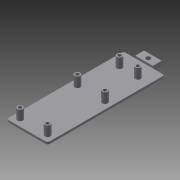
# Autodesk Inventor part: NodeMCU_MQ-7_bottom_v0.2
Saved by Autodesk Inventor 2014 SP1 (Build 180222100, 222)
## iProperties
Created: 2016-10-23
Part Number: NodeMCU_MQ-7_bottom_v0.2
Material: Generic
Document SubType Name: Modeling
Designer: danielsikar
Density: 1 g/cm^3
Appearance: Default
Author: danielsikar
Autodesk Inventor part; units mm, degrees
ref_plane "YZ Plane" through (0, 0, 0) normal (1, 0, 0) x (0, 1, 0)
ref_plane "XZ Plane" through (0, 0, 0) normal (0, 1, 0) x (-1, 0, 0)
ref_plane "XY Plane" through (0, 0, 0) normal (0, 0, 1) x (1, 0, 0)
sketch "Sketch3" plane through (0, 0, 0) normal (0, 0, 1) x (1, 0, 0)
  line L0 (0, 0) -> (37, 0)
  line L1 (37, 0) -> (37, 105.5)
  line L2 (37, 105.5) -> (0, 105.5)
  line L3 (0, 105.5) -> (0, 0)
  dimension "d5" = 37
  dimension "d6" = 105.5
  constraints: 8 end point, 2 parallel, 1 horizontal, 1 perpendicular
  measures "d5" distance of L2.end L1.end
  measures "d6" distance of L1.end L0.end
extrude "Extrusion2" add sketch "Sketch3" along normal blind 2
fillet "Fillet1" radius 2 4 edges at (0, 0, 1) (37, 0, 1) (37, 105.5, 1) (0, 105.5, 1)
sketch "Sketch5" plane through (0, 0, 2) normal (0, 0, 1) x (1, 0, 0)
  line L0 (2, 101.5) -> (2, 4) projected
  line L1 (4, 2) -> (33, 2) projected
  circle A0 centre (6.1, 6.1) radius 2.5
  circle A1 centre (6.1, 6.1) radius 1.5
  line L2 (0, 103.5) -> (0, 2) projected
  line L3 (2, 0) -> (35, 0) projected
  circle A2 centre (6.1, 57.9) radius 2.5
  circle A3 centre (6.1, 57.9) radius 1.5
  circle A4 centre (30.9, 6.1) radius 2.5
  circle A5 centre (30.9, 6.1) radius 1.5
  circle A6 centre (30.9, 57.9) radius 2.5
  circle A7 centre (30.9, 57.9) radius 1.5
  circle A8 centre (10.25, 91.7) radius 2.5
  circle A9 centre (10.25, 91.7) radius 1.5
  circle A10 centre (26.75, 91.7) radius 2.5
  circle A11 centre (26.75, 91.7) radius 1.5
  point P0 (0, 0)
  dimension "d15" = 5
  dimension "d16" = 3
  dimension "d17" = 6.1
  dimension "d18" = 6.1
  dimension "d21" = 51.8
  dimension "d24" = 24.8
  dimension "d27" = 5
  dimension "d28" = 33.8
  dimension "d29" = 4.15
  dimension "d30" = 3
  dimension "d31" = 5
  dimension "d32" = 16.5
  dimension "d33" = 3
  constraints: 12 centre point, 6 coincident, 1 horizontal, 1 vertical, 12 other
  measures "d15" diameter of A0
  measures "d16" diameter of A1
  measures "d17" distance from line of A1.centre L2
  measures "d18" distance from line of A0.centre L3
  measures "d21" distance of A0.centre A2.centre
  measures "d24" distance of A0.centre A4.centre
  measures "d27" diameter of A8
  measures "d28" vertical distance of A8.centre A2.centre
  measures "d29" horizontal distance of A8.centre A2.centre
  measures "d30" diameter of A9
  measures "d31" diameter of A10
  measures "d32" distance of A10.centre A8.centre
  measures "d33" diameter of A11
extrude "Extrusion4" add sketch "Sketch5" along normal blind 9
sketch "Sketch6" plane through (2, 105.5, 0) normal (0, 1, 0) x (1, 0, 0)
  line L0 (33, 0) -> (0, 0) projected
  line L1 (8.5, 0) -> (24.5, 0)
  line L2 (24.5, 0) -> (24.5, -4)
  line L3 (24.5, -4) -> (8.5, -4)
  line L4 (8.5, -4) -> (8.5, 0)
  line L5 (-2, 0) -> (-2, -2) projected
  point P0 (-2, -11)
  dimension "d37" = 16
  dimension "d38" = 4
  dimension "d39" = 10.5
  constraints: 8 end point, 2 parallel, 1 horizontal, 1 perpendicular, 1 point on line
  measures "d37" distance of L2.end L3.end
  measures "d38" distance of L1.end L2.end
  measures "d39" distance from line of L3.end L5
extrude "Extrusion5" add sketch "Sketch6" along normal blind 8
sketch "Sketch7" plane through (7.5, 105.5, 4) normal (0, 0, 1) x (1, 0, 0)
  circle A0 centre (11, 4) radius 2
  line L0 (3, 0) -> (3, 8) projected
  point P0 (-7.5, -105.5)
  point P1 (3, 5)
  point P2 (3, 3)
  dimension "d43" = 4
  dimension "d62" = 8
  constraints: 1 centre point
  measures "d43" diameter of A0
  measures "d62" distance from line of A0.centre L0
extrude "Extrusion6" cut sketch "Sketch7" against normal blind 4
sketch "Sketch9" plane through (0, 0, 2) normal (0, 0, 1) x (1, 0, 0)
  arc A0 (33.4, 6.1) -> (33.4, 6.1) centre (30.9, 6.1) ccw projected
  arc A1 (33.4, 57.9) -> (33.4, 57.9) centre (30.9, 57.9) ccw projected
  arc A2 (8.6, 57.9) -> (8.6, 57.9) centre (6.1, 57.9) ccw projected
  arc A3 (8.6, 6.1) -> (8.6, 6.1) centre (6.1, 6.1) ccw projected
  circle A4 centre (10.25, 91.7) radius 2.5 projected
  circle A5 centre (26.75, 91.7) radius 2.5 projected
  circle A6 centre (6.1, 57.9) radius 1.5
  circle A7 centre (30.9, 57.9) radius 1.5
  circle A8 centre (26.75, 91.7) radius 1.5
  circle A9 centre (10.25, 91.7) radius 1.5
  circle A10 centre (6.1, 6.1) radius 1.5
  circle A11 centre (30.9, 6.1) radius 1.5
  point P0 (0, 0)
  dimension "d51" = 3
  dimension "d52" = 3
  dimension "d53" = 3
  dimension "d54" = 3
  dimension "d55" = 3
  dimension "d56" = 3
  constraints: 6 centre point, 6 coincident
  measures "d51" diameter of A6
  measures "d52" diameter of A7
  measures "d53" diameter of A8
  measures "d54" diameter of A9
  measures "d55" diameter of A10
  measures "d56" diameter of A11
extrude "Extrusion8" cut sketch "Sketch9" against normal blind 2 contours A6 | A7 | A8 | A9 | A10 | A11
chamfer "Chamfer1" distance 2 angle 45 6 edges at (8.75, 91.7, 0) (25.25, 91.7, 0) (29.4, 57.9, 0) (4.6, 57.9, 0) (29.4, 6.1, 0) (4.6, 6.1, 0)
body "Solid2"
